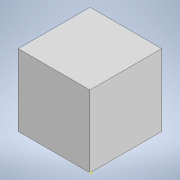
# Autodesk Inventor part: pawn
Saved by Autodesk Inventor 2021 (Build 250183000, 183)
## iProperties
Created: 2021-01-10
Part Number: pawn
Material: Generic
Document SubType Name: Modeling
Designer: Luke Kamols
Density: 1 g/cm^3
Appearance: Default
Author: Luke Kamols
Autodesk Inventor part; units mm, degrees
ref_plane "YZ Plane" through (0, 0, 0) normal (1, 0, 0) x (0, 1, 0)
ref_plane "XZ Plane" through (0, 0, 0) normal (0, 1, 0) x (-1, 0, 0)
ref_plane "XY Plane" through (0, 0, 0) normal (0, 0, 1) x (1, 0, 0)
sketch "Sketch1" plane through (0, 0, 0) normal (0, 1, 0) x (-1, 0, 0)
  point P0 (0, 0)
sketch "Sketch2" plane through (0, 0, 0) normal (0, 1, 0) x (-1, 0, 0)
  line L0 (0, 0) -> (16, 0)
  line L1 (16, 0) -> (16, -16)
  line L2 (16, -16) -> (0, -16)
  line L3 (0, -16) -> (0, 0)
  line L4 (0, 0) -> (0, -8)
  dimension "d1" = 16
  dimension "d2" = 16
  constraints: 10 end point, 2 parallel, 1 horizontal, 1 midpoint, 1 perpendicular
  measures "d1" distance of L1.end L2.end
  measures "d2" distance of L0.end L1.end
extrude "Extrusion1" add sketch "Sketch2" along normal blind 16
sketch "Sketch3" plane through (0, 0, 0) normal (0, -1, 0) x (1, 0, 0)
  line L0 (-16, 0) -> (0, 0) projected
  line L1 (-16, -16) -> (-16, 0) projected
  line L2 (0, 0) -> (0, -16) projected
  line L3 (-1.8, -8) -> (-1.8, -10.2)
  line L4 (-1.8, -10.2) -> (-14.2, -10.2)
  line L5 (-14.2, -10.2) -> (-14.2, -5.8)
  line L6 (-14.2, -5.8) -> (-1.8, -5.8)
  line L7 (-1.8, -5.8) -> (-1.8, -8)
  line L8 (-8, -14.2) -> (-10.2, -14.2)
  line L9 (-10.2, -14.2) -> (-10.2, -1.8)
  line L10 (-10.2, -1.8) -> (-5.8, -1.8)
  line L11 (-5.8, -1.8) -> (-5.8, -14.2)
  line L12 (-5.8, -14.2) -> (-8, -14.2)
  point P0 (-5.8, -5.8)
  point P1 (-10.2, -5.8)
  point P2 (-10.2, -10.2)
  point P3 (-5.8, -10.2)
  dimension "d11" = 2.2
  dimension "d12" = 12.4
  dimension "d13" = 4.4
  dimension "d15" = 2.2
  dimension "d16" = 12.4
  dimension "d17" = 4.4
  constraints: 20 end point, 7 perpendicular, 2 point on line, 1 parallel
  measures "d11" distance of L3.start L3.end
  measures "d12" distance of L3.end L4.end
  measures "d13" distance of L4.end L5.end
  measures "d15" distance of L8.start L8.end
  measures "d16" distance of L8.end L9.end
  measures "d17" distance of L9.end L10.end
extrude "Extrusion2" cut sketch "Sketch3" against normal blind 13
body "Solid1"
